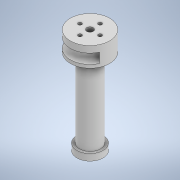
# Autodesk Inventor part: Rotating1inPart
Saved by Autodesk Inventor 2020.3 (Build 243373000, 373)
## iProperties
Created: 2021-03-22
Part Number: Rotating1inPart
Material: Generic
Document SubType Name: Modeling
Designer: tdmp4
Density: 1 g/cm^3
Appearance: Default
Author: tdmp4
Autodesk Inventor part; units mm, degrees
ref_plane "YZ Plane" through (0, 0, 0) normal (1, 0, 0) x (0, 1, 0)
ref_plane "XZ Plane" through (0, 0, 0) normal (0, 1, 0) x (-1, 0, 0)
ref_plane "XY Plane" through (0, 0, 0) normal (0, 0, 1) x (1, 0, 0)
sketch "Sketch1" plane through (0, 0, 0) normal (0, 1, 0) x (-1, 0, 0)
  circle A0 centre (0, 0) radius 10.16
  dimension "d0" = 20.32
  constraints: 1 centre point, 1 coincident
  measures "d0" diameter of A0
extrude "Extrusion1" add sketch "Sketch1" along normal blind 76.2
sketch "Sketch2" plane through (0, 76.2, 0) normal (0, 1, 0) x (1, 0, 0)
  circle A0 centre (0, 0) radius 19.05
  dimension "d3" = 38.1
  constraints: 1 centre point, 1 coincident
  measures "d3" diameter of A0
extrude "Extrusion2" add sketch "Sketch2" along normal blind 12.7
sketch "Sketch6" plane through (0, 88.9, 0) normal (0, 1, 0) x (1, 0, 0)
  arc A0 (17.272, 0) -> (-17.272, 0) centre (0, 0) ccw
  line L0 (17.272, 0) -> (17.272, -8.0362)
  circle A1 centre (0, 0) radius 19.05 projected
  line L1 (-17.272, 0) -> (-17.272, -8.5424)
  line L2 (17.272, -8.0362) -> (17.272, -33.241)
  line L3 (17.272, -33.241) -> (-17.272, -33.241)
  line L4 (-17.272, -33.241) -> (-17.272, -8.5424)
  dimension "d14" = 34.544
  constraints: 10 end point, 3 vertical, 2 perpendicular, 2 point on circle, 1 centre point, 1 coincident, 2 other
  measures "d14" diameter of A0
extrude "Extrusion5" cut sketch "Sketch6" against normal blind 9.525 contours L0 A1 L1 A0 | L2 L3 L4 L1 A1 picked at (0, -6.35)
sketch "Sketch7" plane through (0, 88.9, 0) normal (0, 1, 0) x (1, 0, 0)
  circle A0 centre (0, 0) radius 19.05
  constraints: 1 centre point, 1 coincident
extrude "Extrusion6" add sketch "Sketch7" along normal blind 6.35
sketch "Sketch8" plane through (0, 95.25, 0) normal (0, 1, 0) x (1, 0, 0)
  circle A0 centre (0, 0) radius 9.779
  circle A1 centre (9.779, 0) radius 1.778
  circle A2 centre (0, -9.779) radius 1.778
  circle A3 centre (-9.779, 0) radius 1.778
  circle A4 centre (0, 9.779) radius 1.778
  dimension "d19" = 19.558
  dimension "d20" = 3.556
  dimension "d21" = 3.556
  dimension "d22" = 3.556
  dimension "d23" = 3.556
  constraints: 5 centre point, 4 point on circle, 1 coincident
  measures "d19" diameter of A0
  measures "d20" diameter of A1
  measures "d21" diameter of A2
  measures "d22" diameter of A3
  measures "d23" diameter of A4
extrude "Extrusion7" cut sketch "Sketch8" against normal blind 6.35 contours A0 A1 | A0 A1 | A4 A0 | A0 A4 | A2 A0 | A0 A2 | A3 A0 | A0 A3
sketch "Sketch9" plane through (0, 95.25, 0) normal (0, 1, 0) x (1, 0, 0)
  circle A0 centre (0, 0) radius 10.16 projected
  circle A1 centre (0, 0) radius 3.2004
  dimension "d26" = 6.4008
  constraints: 1 centre point, 1 coincident
  measures "d26" diameter of A1
extrude "Extrusion8" cut sketch "Sketch9" against normal through all contours A1
sketch "Sketch10" plane through (0, 0, 0) normal (0, -1, 0) x (1, 0, 0)
  circle A0 centre (0, 0) radius 12.7
  circle A1 centre (0, 0) radius 3.2004
  dimension "d29" = 25.4
  constraints: 2 centre point, 2 coincident
  measures "d29" diameter of A0
extrude "Extrusion9" add sketch "Sketch10" along normal blind 6.35
body "Solid1"
